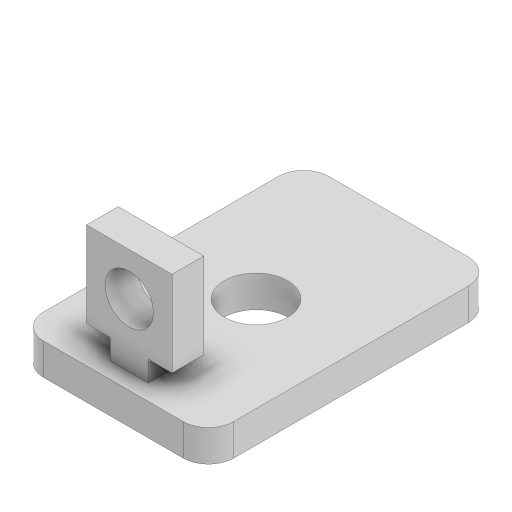
# Autodesk Inventor part: BASE DE YUGO ESCOCES
Saved by Autodesk Inventor 2024 (Build 280153000, 153)
## iProperties
Created: 2024-06-30
Part Number: BASE DE YUGO ESCOCES
Material: Generic
Document SubType Name: Modeling
Designer: Jhuliams
Density: 1 g/cm^3
Appearance: Default
Author: Jhuliams
Autodesk Inventor part; units mm, degrees
ref_plane "YZ Plane" through (0, 0, 0) normal (1, 0, 0) x (0, 1, 0)
ref_plane "XZ Plane" through (0, 0, 0) normal (0, 1, 0) x (-1, 0, 0)
sketch "Sketch1" plane through (0, 0, 0) normal (0, 1, 0) x (-1, 0, 0)
  line L0 (30, 45) -> (-30, 45)
  line L1 (-30, 45) -> (-30, -45)
  line L2 (-30, -45) -> (30, -45)
  line L3 (30, -45) -> (30, 45)
  line L4 (30, 45) -> (-30, -45) construction
  line L5 (-30, 45) -> (30, -45) construction
  point P0 (0, 0)
  dimension "d0" = 60
  dimension "d1" = 90
  constraints: 12 end point, 2 midpoint, 2 parallel, 1 horizontal, 1 perpendicular
  measures "d0" distance of L2.end L1.end
  measures "d1" distance of L1.end L0.end
extrude "Extrusion1" add sketch "Sketch1" along normal blind 10
ref_plane "Work Plane1" through (0, 0, 40) normal (0, 0, 1) x (1, 0, 0)
sketch "Sketch4" plane through (0, 0, 40) normal (0, 0, 1) x (1, 0, 0)
  line L0 (-30, 10) -> (30, 10) projected
  line L1 (0, 10) -> (0, 30)
  line L2 (-5, 10) -> (5, 10)
  circle A0 centre (0, 30) radius 7.6
  line L3 (-13.5, 43.5) -> (13.5, 43.5)
  line L4 (13.5, 43.5) -> (13.5, 16.5)
  line L5 (13.5, 16.5) -> (-13.5, 16.5)
  line L6 (-13.5, 16.5) -> (-13.5, 43.5)
  line L7 (-13.5, 43.5) -> (13.5, 16.5) construction
  line L8 (13.5, 43.5) -> (-13.5, 16.5) construction
  line L9 (-6, 18) -> (6, 18)
  line L10 (6, 18) -> (6, 2)
  line L11 (6, 2) -> (-6, 2)
  line L12 (-6, 2) -> (-6, 18)
  line L13 (-6, 18) -> (6, 2) construction
  line L14 (6, 18) -> (-6, 2) construction
  point P0 (0, 0)
  point P1 (6, 16.5)
  point P2 (-6, 16.5)
  dimension "d11" = 20
  dimension "d27" = 15.2
  dimension "d28" = 27
  dimension "d29" = 27
  dimension "d30" = 12
  dimension "d31" = 16
  constraints: 28 end point, 5 midpoint, 4 parallel, 2 horizontal, 2 perpendicular, 1 centre point, 1 coincident, 1 vertical
  measures "d11" distance of L1.start L1.end
  measures "d27" diameter of A0
  measures "d28" distance of L4.end L5.end
  measures "d29" distance of L3.end L4.end
  measures "d30" distance of L10.end L11.end
  measures "d31" distance of L9.end L10.end
extrude "Extrusion3" add sketch "Sketch4" against normal blind 10
fillet "Fillet2" radius 8 4 edges at (-30, 5, 45) (30, 5, 45) (30, 5, -45) (-30, 5, -45)
sketch "Sketch5" plane through (0, 10, 0) normal (0, 1, 0) x (1, 0, 0)
  circle A0 centre (0, 0) radius 10
  dimension "d20" = 20
  constraints: 1 centre point, 1 coincident
  measures "d20" diameter of A0
extrude "Extrusion4" cut sketch "Sketch5" against normal blind 10
sketch "Sketch6" plane through (0, 0, 40) normal (0, 0, 1) x (1, 0, 0)
  point P0 (0, 0)
sketch "Sketch7" plane through (0, 0, 40) normal (0, 0, 1) x (1, 0, 0)
  point P0 (0, 0)
body "Solid1"
